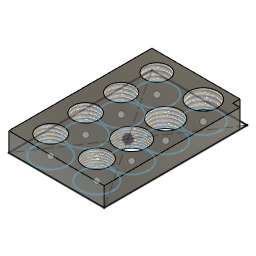
ButtonHoleChecker (Autodesk Fusion 360 design; units mm, degrees)
Autodesk Fusion 360 part; units mm, degrees
sketch "Sketch3" plane through (0, 0, 0) normal (0, 0, 1) x (1, 0, 0)
  line L0 (10, 15) -> (-10, 15)
  line L1 (-10, 15) -> (-10, -15)
  line L2 (-10, -15) -> (10, -15)
  line L3 (10, -15) -> (10, 15)
  line L4 (10, 15) -> (-10, -15) construction
  line L5 (-10, 15) -> (10, -15) construction
  circle A0 centre (-5.1854, -3.7051) radius 3.5
  circle A1 centre (4.3644, -3.6049) radius 3.5
  circle A2 centre (-5.0469, -11.1711) radius 3.5
  circle A3 centre (4.3207, -10.8626) radius 3.5
  circle A4 centre (-5.1568, 3.7146) radius 3.5
  circle A5 centre (4.2608, 3.6364) radius 3.5
  circle A6 centre (-5.0509, 11.1009) radius 3.5
  circle A7 centre (4.7212, 11.0813) radius 3.5
  dimension "d22" = 20
  dimension "d23" = 30
  dimension "d24" = 7
  dimension "d25" = 7
  dimension "d26" = 7
  dimension "d27" = 7
  dimension "d34" = 7
  dimension "d35" = 7
  dimension "d36" = 7
  dimension "d37" = 7
  constraint horizontal L0
  constraint perpendicular L0 L1
  constraint parallel L0 L2
  constraint parallel L1 L3
  constraint coincident L4 origin
  constraint coincident L5 origin
  measures "d22" distance of L1.end L2.end
  measures "d23" distance of L0.end L1.end
  measures "d24" diameter of A0
  measures "d25" diameter of A1
  measures "d26" diameter of A2
  measures "d27" diameter of A3
  measures "d34" diameter of A4
  measures "d35" diameter of A5
  measures "d36" diameter of A6
  measures "d37" diameter of A7
extrude "Extrude6" add sketch "Sketch3" along normal blind 4
sketch "Sketch5" plane through (0, 0, 4) normal (0, 0, 1) x (-1, 0, 0)
  circle A0 centre (5.1854, 3.7051) radius 3.5
  circle A1 centre (5.0469, 11.1711) radius 3.5
  circle A2 centre (-4.3644, 3.6049) radius 3.5
  circle A3 centre (-4.3207, 10.8626) radius 3.5
  circle A4 centre (5.1568, -3.7146) radius 3.5
  circle A5 centre (-4.2608, -3.6364) radius 3.5
  circle A6 centre (5.0509, -11.1009) radius 3.5
  circle A7 centre (-4.7212, -11.0813) radius 3.5
  line L0 (-10, 15) -> (-10, -15)
  line L1 (-10, -15) -> (10, -15)
  line L2 (10, -15) -> (10, 15)
  line L3 (10, 15) -> (-10, 15)
  line L4 (-10, -15) -> (-8.5, -15)
  line L5 (-8.5, -15) -> (-8.5, -13.5)
  line L6 (-8.5, -13.5) -> (-10, -13.5)
  line L7 (-10, -13.5) -> (-10, -15)
  dimension "d40" = 1.5
  dimension "d41" = 1.5
  constraint horizontal L4
  constraint vertical L5
  constraint horizontal L6
  constraint vertical L7
  constraint coincident L0.end L1.start
  measures "d40" distance of L0.end L4.end
  measures "d41" distance of L0.end L6.end
extrude "Extrude7" cut sketch "Sketch5" against normal blind 4 contours L0 L1 L4 L5 L6 L7
thread "Thread6" "ISO Metric profile 6.0 M6x1 6H" major diameter 6.147 minor diameter 5.035 pitch 1 angle 60 resizes the face on face at (-1.5553, 10.9264, 2.6667)
thread "Thread7" "ISO Metric profile 6.0 M6x0.8 6H" major diameter 6.1107 minor diameter 5.234 pitch 0.8 angle 60 resizes the face on face at (-1.6611, 3.8891, 1.3333)
thread "Thread8" "ISO Metric profile 6.0 M6x0.75 6H" major diameter 6.1201 minor diameter 5.2831 pitch 0.75 angle 60 resizes the face on face at (-1.6898, -3.5307, 1.3333)
thread "Thread9" "ISO Metric profile 6.0 M6x0.7 6H" major diameter 6.1132 minor diameter 5.3322 pitch 0.7 angle 60 resizes the face on face at (-1.5513, -10.9966, 1.3333)
thread "Thread10" "ISO Metric profile 7.0 M7x1 6H" major diameter 7.1472 minor diameter 6.0355 pitch 1 angle 60 resizes the face on face at (8.2169, 11.2557, 1.3333)
thread "Thread11" "ISO Metric profile 7.0 M7x0.75 6H" major diameter 7.1201 minor diameter 6.2831 pitch 0.75 angle 60 resizes the face on face at (7.7565, 3.8108, 1.3333)
thread "Thread12" "ISO Metric profile 7.0 M7x0.5 6H" major diameter 7.0922 minor diameter 6.5287 pitch 0.5 angle 60 resizes the face on face at (7.86, -3.4304, 1.3333)
thread "Thread13" "ISO Metric profile 6.0 M6x0.5 6H" major diameter 6.0922 minor diameter 5.5287 pitch 0.5 angle 60 resizes the face on face at (7.8163, -10.6881, 1.3333)
